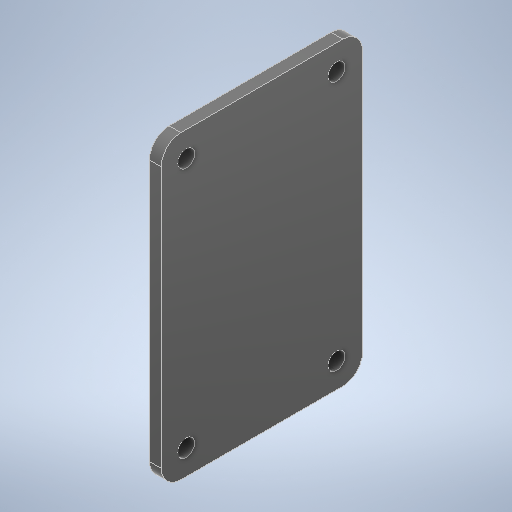
# Autodesk Inventor part: Rotary Actuator Platform Design 2
Saved by Autodesk Inventor 2025.1 (Build 291241020, 241B)
## iProperties
Company: 1P13
RuleStatus: InUse
Created: 2024-05-09
Part Number: Rotary Actuator Platform Design 2
Material: Acetal Resin, Black
Document SubType Name: Modeling
Designer: A 1P13 IAI
Density: 1.425 g/cm^3
Appearance: Smooth - Black
User Status: Plain
AfterDocOpen0: OpenForm
Author: A 1P13 IAI
Title: 1P13 Modular Plane Part
Autodesk Inventor part; units mm, degrees
sketch "Body Sketch" plane through (0, 0, 0) normal (1, 0, 0) x (0, 1, 0)
  line L0 (0, 0) -> (76.2, 0)
  line L1 (76.2, 0) -> (76.2, -51.05)
  line L2 (76.2, -51.05) -> (0, -51.05)
  line L3 (0, -51.05) -> (0, 0)
  dimension "d2" = 76.2
  dimension "d3" = 51.05
  constraints: 8 end point, 2 parallel, 1 horizontal, 1 perpendicular
  measures "d2" distance of L0.start L0.end
  measures "d3" distance of L2.end L0.start
extrude "Body Extrude" add sketch "Body Sketch" along normal blind 3
ref_plane "Work Plane1" through (0, 38.1, -51.05) normal (0, -1, 0) x (1, 0, 0)
ref_plane "Work Plane2" through (0, 0, -25.525) normal (0, 0, 1) x (1, 0, 0)
ref_plane "Work Plane3" through (0, 0, 0) normal (0, -0.7071, -0.7071) x (1, 0, 0)
ref_plane "Work Plane4" through (0, 76.2, 0) normal (0, 0.7071, -0.7071) x (-1, 0, 0)
sketch "Hole Sketch" plane through (3, 0, 0) normal (1, 0, 0) x (0, 0, -1)
  line L0 (0, 0) -> (6.35, 0) construction
  line L1 (6.35, 0) -> (6.35, 6.35) construction
  line L2 (6.35, 6.35) -> (0, 6.35) construction
  line L3 (0, 6.35) -> (0, 0) construction
  point P0 (44.45, 6.35)
  point P1 (-19.2059, 16.3555)
  point P2 (6.35, 69.85)
  point P3 (44.45, 69.85)
  dimension "d4" = 6.35
  dimension "d55" = 38.1
  dimension "d56" = 63.5
  constraints: 8 end point, 2 horizontal alignment, 2 parallel, 2 perpendicular, 2 vertical alignment, 1 coincident, 1 horizontal
  measures "d4" distance of L2.end L0.start
  measures "d55" distance of point (44.45, 6.35) L1.end
  measures "d56" distance of point (6.35, 6.35) point (6.35, 69.85)
hole "Hole" at (3, 6.35, -6.35) at (3, 69.85, -6.35) at (3, 69.85, -44.45) at (3, 6.35, -44.45) direction (-1, 0, 0) diameter 4.25 end through all
fillet "Fillet2" radius 5 4 edges at (1.5, 76.2, 0) (1.5, 0, 0) (1.5, 76.2, -51.05) (1.5, 0, -51.05)
equation "\"d54\" = FilletRadius"
equation "\"d4\" = 0.5 * GridSpacing"
equation "\"d5\" = HoleDiam"
equation "\"Thickness\" = 3"
equation "\"GridSpacing\" = 12.7"
equation "\"HoleDiam\" = 4.25"
equation "\"FilletRadius\" = 5"
body "Solid1"
